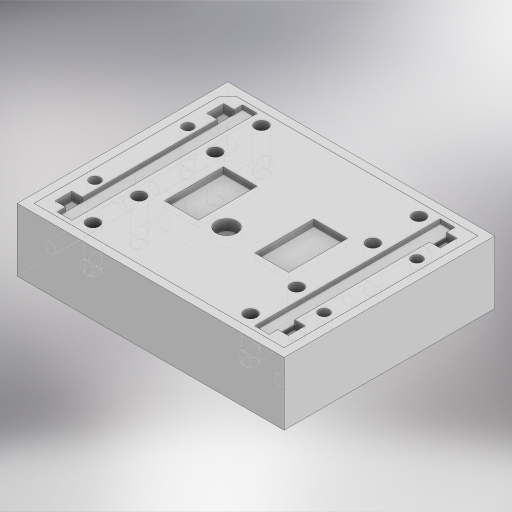
# Autodesk Inventor part: Suction Stage
Saved by Autodesk Inventor 2024 (Build 280153000, 153)
## iProperties
Created: 2024-01-02
Part Number: Suction Stage
Material: Generic
Document SubType Name: Modeling
Designer: cfang
Density: 1 g/cm^3
Appearance: Default
Author: cfang
Autodesk Inventor part; units mm, degrees
ref_plane "YZ Plane" through (0, 0, 0) normal (1, 0, 0) x (0, 1, 0)
ref_plane "XZ Plane" through (0, 0, 0) normal (0, 1, 0) x (-1, 0, 0)
ref_plane "XY Plane" through (0, 0, 0) normal (0, 0, 1) x (1, 0, 0)
sketch "Sketch1" plane through (0, 0, 0) normal (0, 1, 0) x (-1, 0, 0)
  line L0 (-31.75, -25.05) -> (31.75, -25.05)
  line L1 (31.75, -25.05) -> (31.75, 25.05)
  line L2 (31.75, 25.05) -> (-31.75, 25.05)
  line L3 (-31.75, 25.05) -> (-31.75, -25.05)
  line L4 (-31.75, -25.05) -> (31.75, 25.05) construction
  line L5 (31.75, -25.05) -> (-31.75, 25.05) construction
  point P0 (0, 0)
  dimension "d0" = 50.1
  dimension "d1" = 63.5
  constraints: 12 end point, 2 midpoint, 2 parallel, 1 horizontal, 1 perpendicular
  measures "d0" distance of L0.end L1.end
  measures "d1" distance of L1.end L2.end
extrude "Extrusion1" add sketch "Sketch1" along normal blind 15
sketch "Sketch2" plane through (0, 15, 0) normal (0, 1, 0) x (1, 0, 0)
  line L0 (29.75, 23.05) -> (-29.75, 23.05)
  line L1 (-29.75, 23.05) -> (-29.75, -23.05)
  line L2 (-29.75, -23.05) -> (29.75, -23.05)
  line L3 (29.75, -23.05) -> (29.75, 23.05)
  line L4 (29.75, 23.05) -> (-29.75, -23.05) construction
  line L5 (-29.75, 23.05) -> (29.75, -23.05) construction
  line L6 (-29.75, 21.05) -> (-27.75, 23.05)
  line L7 (-29.75, 21.05) -> (-26.9216, 21.05) construction
  point P0 (0, 0)
  dimension "d4" = 46.1
  dimension "d5" = 59.5
  dimension "d6" = 45
  dimension "d7" = 2
  constraints: 16 end point, 2 horizontal, 2 midpoint, 2 parallel, 2 point on line, 1 equal length, 1 perpendicular
  measures "d4" distance of L0.end L1.end
  measures "d5" distance of L1.end L2.end
  measures "d6" angle of L7 L6
  measures "d7" horizontal distance of L6.start L6.end
extrude "Extrusion2" cut sketch "Sketch2" against normal blind 0.011 contours L3 L2 L1 L6 L0
sketch "Sketch3" plane through (0, 14.989, 0) normal (0, 1, 0) x (1, 0, 0)
  line L0 (-27.75, -20.05) -> (-25.25, -20.05)
  line L1 (-25.25, -20.05) -> (-25.25, -16.05)
  line L2 (-25.25, -16.05) -> (-27.75, -16.05)
  line L3 (-27.75, -16.05) -> (-27.75, -20.05)
  line L4 (29.75, -23.05) -> (-29.75, -23.05) projected
  line L5 (-29.75, -23.05) -> (-29.75, 21.05) projected
  line L6 (-25.25, 16.05) -> (-27.75, 16.05)
  line L7 (-27.75, 16.05) -> (-27.75, 20.05)
  line L8 (-27.75, 20.05) -> (-25.25, 20.05)
  line L9 (-25.25, 20.05) -> (-25.25, 16.05)
  line L10 (-27.75, 23.05) -> (29.75, 23.05) projected
  line L11 (25.25, -20.05) -> (27.75, -20.05)
  line L12 (27.75, -20.05) -> (27.75, -16.05)
  line L13 (27.75, -16.05) -> (25.25, -16.05)
  line L14 (25.25, -16.05) -> (25.25, -20.05)
  line L15 (25.25, 16.05) -> (27.75, 16.05)
  line L16 (27.75, 16.05) -> (27.75, 20.05)
  line L17 (27.75, 20.05) -> (25.25, 20.05)
  line L18 (25.25, 20.05) -> (25.25, 16.05)
  line L19 (29.75, 23.05) -> (29.75, -23.05) projected
  point P0 (0, 0)
  point P1 (26.5, -20.05)
  point P2 (26.5, -16.05)
  dimension "d10" = 3
  dimension "d11" = 7
  dimension "d12" = 2
  dimension "d13" = 4.5
  dimension "d14" = 2
  dimension "d15" = 3
  dimension "d16" = 7
  dimension "d17" = 4.5
  dimension "d18" = 3
  dimension "d19" = 2
  dimension "d20" = 7
  dimension "d21" = 4.5
  dimension "d22" = 3
  dimension "d23" = 7
  dimension "d24" = 2
  dimension "d25" = 4.5
  constraints: 32 end point, 8 parallel, 4 horizontal, 4 perpendicular, 2 midpoint
  measures "d10" distance between parallel lines of L4 L0
  measures "d11" distance between parallel lines of L4 L2
  measures "d12" distance between parallel lines of L3 L5
  measures "d13" distance between parallel lines of L5 L1
  measures "d14" distance between parallel lines of L5 L7
  measures "d15" distance between parallel lines of L10 L8
  measures "d16" distance between parallel lines of L10 L6
  measures "d17" distance between parallel lines of L9 L5
  measures "d18" distance from line of L4 point (26.5, -20.05)
  measures "d19" distance between parallel lines of L19 L12
  measures "d20" distance from line of L4 point (26.5, -16.05)
  measures "d21" distance between parallel lines of L19 L14
  measures "d22" distance between parallel lines of L10 L17
  measures "d23" distance between parallel lines of L10 L15
  measures "d24" distance between parallel lines of L16 L19
  measures "d25" distance between parallel lines of L18 L19
extrude "Extrusion3" cut sketch "Sketch3" against normal blind 2
sketch "Sketch4" plane through (0, 14.989, 0) normal (0, 1, 0) x (1, 0, 0)
  line L0 (21.75, 22.05) -> (25.25, 22.05)
  line L1 (25.25, 22.05) -> (25.25, -22.05)
  line L2 (25.25, -22.05) -> (21.75, -22.05)
  line L3 (21.75, -22.05) -> (21.75, 22.05)
  line L4 (29.75, 23.05) -> (29.75, -23.05) projected
  line L5 (-27.75, 23.05) -> (29.75, 23.05) projected
  line L6 (29.75, -23.05) -> (-29.75, -23.05) projected
  line L7 (-21.75, -22.05) -> (-25.25, -22.05)
  line L8 (-25.25, -22.05) -> (-25.25, 22.05)
  line L9 (-25.25, 22.05) -> (-21.75, 22.05)
  line L10 (-21.75, 22.05) -> (-21.75, -22.05)
  line L11 (-29.75, -23.05) -> (-29.75, 21.05) projected
  point P0 (0, 0)
  dimension "d28" = 4.5
  dimension "d29" = 8
  dimension "d30" = 1
  dimension "d31" = 1
  dimension "d34" = 1
  dimension "d35" = 1
  dimension "d36" = 4.5
  dimension "d37" = 8
  constraints: 16 end point, 4 parallel, 2 horizontal, 2 perpendicular
  measures "d28" distance between parallel lines of L1 L4
  measures "d29" distance between parallel lines of L4 L3
  measures "d30" distance between parallel lines of L5 L0
  measures "d31" distance between parallel lines of L6 L2
  measures "d34" distance between parallel lines of L5 L9
  measures "d35" distance between parallel lines of L6 L7
  measures "d36" distance between parallel lines of L11 L8
  measures "d37" distance between parallel lines of L10 L11
extrude "Extrusion4" cut sketch "Sketch4" against normal blind 1
sketch "Sketch5" plane through (0, 14.989, 0) normal (0, 1, 0) x (1, 0, 0)
  line L0 (14.75, 7) -> (6.75, 7)
  line L1 (6.75, 7) -> (6.75, -7)
  line L2 (6.75, -7) -> (14.75, -7)
  line L3 (14.75, -7) -> (14.75, 7)
  line L4 (14.75, 7) -> (6.75, -7) construction
  line L5 (6.75, 7) -> (14.75, -7) construction
  line L6 (29.75, 23.05) -> (29.75, -23.05) projected
  line L7 (-6.75, -7) -> (-14.75, -7)
  line L8 (-14.75, -7) -> (-14.75, 7)
  line L9 (-14.75, 7) -> (-6.75, 7)
  line L10 (-6.75, 7) -> (-6.75, -7)
  line L11 (-6.75, -7) -> (-14.75, 7) construction
  line L12 (-14.75, -7) -> (-6.75, 7) construction
  line L13 (-29.75, -23.05) -> (-29.75, 21.05) projected
  point P0 (0, 0)
  point P1 (10.75, 0)
  point P2 (-10.75, 0)
  dimension "d38" = 15
  dimension "d39" = 23
  dimension "d40" = 14
  dimension "d41" = 14
  dimension "d43" = 23
  dimension "d44" = 15
  constraints: 24 end point, 4 midpoint, 4 parallel, 2 horizontal, 2 horizontal alignment, 2 perpendicular
  measures "d38" distance between parallel lines of L6 L3
  measures "d39" distance between parallel lines of L6 L1
  measures "d40" distance of L0.end L1.end
  measures "d41" distance of L7.end L8.end
  measures "d43" distance between parallel lines of L13 L10
  measures "d44" distance between parallel lines of L8 L13
extrude "Extrusion5" cut sketch "Sketch5" against normal blind 1.5
sketch "Sketch6" plane through (0, 14.989, 0) normal (0, 1, 0) x (1, 0, 0)
  circle A0 centre (-1.95, -5.05) radius 2.5
  line L0 (29.75, -23.05) -> (-29.75, -23.05) projected
  line L1 (29.75, 23.05) -> (29.75, -23.05) projected
  point P0 (0, 0)
  dimension "d47" = 5
  dimension "d48" = 18
  dimension "d49" = 31.7
  constraints: 1 centre point
  measures "d47" diameter of A0
  measures "d48" distance from line of L0 A0.centre
  measures "d49" distance from line of L1 A0.centre
extrude "Extrusion6" cut sketch "Sketch6" against normal blind 2.5
sketch "Sketch7" plane through (0, 14.989, 0) normal (0, 1, 0) x (1, 0, 0)
  circle A0 centre (27.25, -11.05) radius 1.25
  circle A1 centre (27.25, 11.05) radius 1.25
  line L0 (29.75, 23.05) -> (29.75, -23.05) projected
  line L1 (-27.75, 23.05) -> (29.75, 23.05) projected
  line L2 (29.75, -23.05) -> (-29.75, -23.05) projected
  circle A2 centre (18.75, 20.05) radius 1.5
  circle A3 centre (18.75, 9.05) radius 1.5
  circle A4 centre (18.75, -9.05) radius 1.5
  circle A5 centre (18.75, -20.05) radius 1.5
  line L3 (0, -18.55) -> (0, 18.55)
  circle A6 centre (-27.25, -11.05) radius 1.25
  circle A7 centre (-27.25, 11.05) radius 1.25
  line L4 (-29.75, 23.05) -> (-29.75, -23.05)
  circle A8 centre (-18.75, 20.05) radius 1.5
  circle A9 centre (-18.75, 9.05) radius 1.5
  circle A10 centre (-18.75, -9.05) radius 1.5
  circle A11 centre (-18.75, -20.05) radius 1.5
  point P0 (0, 0)
  dimension "d52" = 2.5
  dimension "d53" = 2.5
  dimension "d54" = 2.5
  dimension "d55" = 12
  dimension "d56" = 2.5
  dimension "d57" = 12
  dimension "d58" = 3
  dimension "d59" = 3
  dimension "d60" = 3
  dimension "d61" = 3
  dimension "d63" = 3
  dimension "d64" = 3
  dimension "d65" = 11
  dimension "d66" = 11
  dimension "d67" = 11
  constraints: 12 centre point, 7 symmetric about line, 4 end point, 2 vertical alignment, 1 vertical, 6 other
  measures "d52" diameter of A0
  measures "d53" diameter of A1
  measures "d54" distance from line of L0 A1.centre
  measures "d55" distance from line of A1.centre L1
  measures "d56" distance from line of L0 A0.centre
  measures "d57" distance from line of L2 A0.centre
  measures "d58" diameter of A2
  measures "d59" diameter of A3
  measures "d60" diameter of A4
  measures "d61" diameter of A5
  measures "d63" distance from line of L2 A5.centre
  measures "d64" distance from line of A2.centre L1
  measures "d65" distance of A5.centre A4.centre
  measures "d66" distance of A2.centre A3.centre
  measures "d67" distance from line of L0 A5.centre
extrude "Extrusion7" cut sketch "Sketch7" against normal blind 10
sketch "Sketch8" plane through (-31.75, 0, -25.05) normal (-1, 0, 0) x (0, 0, 1)
  line L0 (0, 0) -> (50.1, 0) projected
  point P0 (25.05, 0)
  point P1 (25.05, 6)
  dimension "d70" = 6
  measures "d70" distance from line of L0 point (25.05, 6)
hole "Hole1" at (-31.75, 6, 0) direction (1, 0, 0) diameter 6.35 depth 60
sketch "Sketch10" plane through (-31.75, 0, 25.05) normal (0, 0, 1) x (1, 0, 0)
  circle A0 centre (4.4865, 6.2999) radius 1.25
  circle A1 centre (13.0295, 6.489) radius 1.5
  line L0 (11.5, 4.989) -> (14.5, 4.989) projected
  circle A2 centre (50.5, 6.489) radius 1.5
  line L1 (49, 4.989) -> (52, 4.989) projected
  circle A3 centre (59, 6.239) radius 1.25
  line L2 (57.75, 4.989) -> (60.25, 4.989) projected
  point P0 (31.75, 0)
  dimension "d78" = 2.5
  dimension "d81" = 3
  dimension "d82" = 3
  dimension "d83" = 2.5
  constraints: 4 centre point, 3 tangent
  measures "d78" diameter of A0
  measures "d81" diameter of A1
  measures "d82" diameter of A2
  measures "d83" diameter of A3
extrude "Extrusion8" cut sketch "Sketch10" against normal up to surface (50.1 mm away) from surface at 0
sketch "Sketch11" plane through (-31.75, 0, 25.05) normal (0, 0, 1) x (1, 0, 0)
  circle A0 centre (4.4865, 6.2999) radius 1.25 projected
  circle A1 centre (13.0295, 6.489) radius 1.5 projected
  circle A2 centre (50.5, 6.489) radius 1.5 projected
  circle A3 centre (59, 6.239) radius 1.25 projected
  point P0 (31.75, 0)
extrude "Extrusion9" add sketch "Sketch11" against normal blind 3.5
sketch "Sketch12" plane through (31.75, 0, -25.05) normal (0, 0, -1) x (-1, 0, 0)
  circle A0 centre (4.5, 6.239) radius 1.25 projected
  circle A1 centre (13, 6.489) radius 1.5 projected
  circle A2 centre (50.4705, 6.489) radius 1.5 projected
  circle A3 centre (59.0135, 6.2999) radius 1.25 projected
  point P0 (31.75, 0)
extrude "Extrusion10" add sketch "Sketch12" against normal blind 3.5
equation "\"d14\" = d12"
equation "\"d15\" = d10"
equation "\"d16\" = d11"
equation "\"d17\" = d13"
equation "\"d18\" = d10"
equation "\"d19\" = d12"
equation "\"d20\" = d11"
equation "\"d21\" = d13"
equation "\"d22\" = d15"
equation "\"d23\" = d16"
equation "\"d24\" = d14"
equation "\"d25\" = d17"
equation "\"d41\" = d40"
equation "\"d43\" = d39"
equation "\"d44\" = d38"
equation "\"d56\" = d54"
equation "\"d57\" = d55"
body "Solid1"
